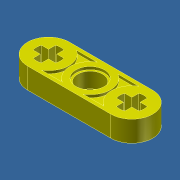
# Autodesk Inventor part: LEGO Brick 32017
Saved by Autodesk Inventor 2011 SP2 (Build 150553200, 553)
## iProperties
Company: Allseas Engineering BV
Created: 2011-11-29
Part Number: LEGO Brick 32017
Cost Center: 0 kg
Material: Steel
Document SubType Name: Modeling
Designer: BvH
Authority: 0 mm^3
Stock Number: =<Filenr>_<Document number>
Density: 7.85 g/cm^3
Mass: 4.0904 g
Surface Area: 7.54331 cm^2
Volume: 0.521071 cm^3
Act. Code: DW000
SaveDate: 2011-07-28
SaveTime: 18:32
FileName: Standard
TotalMass: 0 kg
TotalVolume: 0 mm^3
Subject: =<Title><TITLE 1_2> <TITLE 2_2>
Author: BvH
Autodesk Inventor part; units mm, degrees
ref_plane "YZ Plane" through (0, 0, 0) normal (1, 0, 0) x (0, 1, 0)
ref_plane "XZ Plane" through (0, 0, 0) normal (0, 1, 0) x (-1, 0, 0)
ref_plane "XY Plane" through (0, 0, 0) normal (0, 0, 1) x (1, 0, 0)
sketch "Sketch1" plane through (0, 0, 0) normal (0, 0, 1) x (1, 0, 0)
  line L0 (0, -5.6) -> (0, 5.6) construction
  line L1 (-16.8, 0) -> (16.8, 0) construction
  line L2 (8, 4) -> (-8, 4)
  arc A0 (-8, 4) -> (-8, -4) centre (-8, 0) ccw
  line L3 (-8, -4) -> (8, -4)
  arc A1 (8, -4) -> (8, 4) centre (8, 0) ccw
  circle A2 centre (0, 0) radius 2.75
  circle A3 centre (0, 0) radius 2.4
  point P0 (0, 4)
  dimension "d0" = 24
  dimension "d1" = 8
  dimension "d27" = 4.8
  dimension "d28" = 5.5
  constraints: 4 centre point, 4 end point, 4 point on circle, 4 tangent, 3 midpoint, 2 horizontal, 2 point on line, 1 coincident
  measures "d1" distance between parallel lines of L2 L3
  measures "d27" diameter of A3
  measures "d28" diameter of A2
sketch "Sketch6" plane through (0, 0, 0) normal (0, 0, 1) x (1, 0, 0)
  arc A0 (-8, 4) -> (-8, -4) centre (-8, 0) ccw construction
  arc A1 (8, -4) -> (8, 4) centre (8, 0) ccw construction
  circle A2 centre (-8, 0) radius 2.3
  circle A3 centre (8, 0) radius 2.3
  line L0 (-10.1564, 0.8) -> (-8.8, 0.8)
  line L1 (-8.8, 0.8) -> (-8.8, 2.1564)
  line L2 (-7.2, 2.1564) -> (-7.2, 0.8)
  line L3 (-7.2, 0.8) -> (-5.8436, 0.8)
  line L4 (-5.8436, -0.8) -> (-7.2, -0.8)
  line L5 (-7.2, -0.8) -> (-7.2, -2.1564)
  line L6 (-8.8, -2.1564) -> (-8.8, -0.8)
  line L7 (-8.8, -0.8) -> (-10.1564, -0.8)
  line L8 (5.8436, 0.8) -> (7.2, 0.8)
  line L9 (8.8, 0.8) -> (10.1564, 0.8)
  line L10 (8.8, 2.1564) -> (8.8, 0.8)
  line L11 (8.8, -0.8) -> (8.8, -2.1564)
  line L12 (7.2, 2.1564) -> (7.2, 0.8)
  line L13 (7.2, -0.8) -> (7.2, -2.1564)
  line L14 (10.1564, -0.8) -> (8.8, -0.8)
  line L15 (7.2, -0.8) -> (5.8436, -0.8)
  dimension "d29" = 4.6
  dimension "d30" = 1.6
  constraints: 32 end point, 13 equal length, 8 horizontal, 8 vertical, 2 coincident, 2 collinear, 20 other
  measures "d30" distance between parallel lines of L2 L1
extrude "Extrusion1" add sketch "Sketch1" along normal mid plane 4 contours A1 L3 A0 L2 | A2 | A3
extrude "Extrusion2" cut sketch "Sketch1" along normal through all both and the other way through all contours A3
sketch "Sketch2" plane through (0, 0, 2) normal (0, 0, 1) x (1, 0, 0)
  circle A0 centre (0, 0) radius 2.75 projected
extrude "Extrusion3" cut sketch "Sketch2" against normal blind 0.5333
sketch "Sketch3" plane through (0, 0, -2) normal (0, 0, -1) x (-1, 0, 0)
  circle A0 centre (0, 0) radius 2.75 projected
extrude "Extrusion4" cut sketch "Sketch3" against normal blind 0.5333
extrude "Extrusion7" cut sketch "Sketch6" along normal through all both and the other way through all contours A2 L4 L5 L6 L7 L0 L1 L2 L3 | A3 L14 L11 L13 L15 L8 L12 L10 L9
sketch "Sketch4" plane through (0, 0, 2) normal (0, 0, 1) x (1, 0, 0)
  circle A0 centre (-8, 0) radius 2.3 construction
  circle A1 centre (8, 0) radius 2.3 construction
  arc A2 (5.9892, 3.3333) -> (5.9892, -3.3333) centre (8, 0) ccw
  line L0 (2.0108, 3.3333) -> (5.9892, 3.3333)
  line L1 (5.9892, -3.3333) -> (2.0108, -3.3333)
  arc A3 (-5.9892, -3.3333) -> (-5.9892, 3.3333) centre (-8, 0) ccw
  line L2 (-5.9892, 3.3333) -> (-2.0108, 3.3333)
  line L3 (-5.9892, -3.3333) -> (-2.0108, -3.3333)
  arc A4 (2.0108, -3.3333) -> (2.0108, 3.3333) centre (0, 0) ccw
  arc A5 (-2.0108, 3.3333) -> (-2.0108, -3.3333) centre (0, 0) ccw
  circle A6 centre (0, 0) radius 2.75 construction
  dimension "d33" = 6.6667
  dimension "d35" = 1.1429
  constraints: 8 end point, 8 point on circle, 4 centre point, 4 horizontal, 3 coincident, 3 equal radius, 2 collinear, 1 parallel
  measures "d33" distance between parallel lines of L3 L2
  measures "d35" radial gap between concentric circles of A5 A6
extrude "Extrusion5" cut sketch "Sketch4" against normal blind 0.5333
sketch "Sketch7" plane through (0, 0, -2) normal (0, 0, -1) x (-1, 0, 0)
  arc A0 (5.9892, 3.3333) -> (5.9892, -3.3333) centre (8, 0) ccw projected
  line L0 (5.9892, -3.3333) -> (2.0108, -3.3333) projected
  arc A1 (2.0108, -3.3333) -> (2.0108, 3.3333) centre (0, 0) ccw projected
  line L1 (2.0108, 3.3333) -> (5.9892, 3.3333) projected
  arc A2 (-2.0108, 3.3333) -> (-2.0108, -3.3333) centre (0, 0) ccw projected
  line L2 (-2.0108, -3.3333) -> (-5.9892, -3.3333) projected
  arc A3 (-5.9892, -3.3333) -> (-5.9892, 3.3333) centre (-8, 0) ccw projected
  line L3 (-5.9892, 3.3333) -> (-2.0108, 3.3333) projected
extrude "Extrusion8" cut sketch "Sketch7" against normal blind 0.5333
equation "\"d1\" = width_standard"
equation "\"d2\" = 0.5 * width_standard"
equation "\"d6\" = 0.333333 * height_standard"
equation "\"d13\" = 0.0555556 * height_standard"
equation "\"d15\" = 0.0555556 * height_standard"
equation "\"d33\" = 0.833333 * width_standard"
equation "\"d20\" = 0.0555556 * height_standard"
equation "\"d36\" = 0.0555556 * height_standard"
equation "\"width_standard\" = 8"
equation "\"height_standard\" = 9.6"
body "Solid1"
